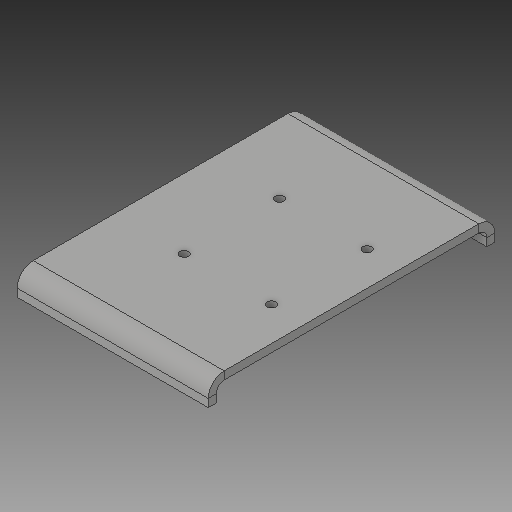
# Autodesk Inventor part: shapeoko_zplate
Saved by Autodesk Inventor 2019 (Build 230136000, 136)
## iProperties
Created: 2017-12-20
Part Number: shapeoko_zplate
Material: Generic
Document SubType Name: Sheet Metal
Designer: MISAKA
Density: 1 g/cm^3
Sheet Metal Rule: Default_mm
Appearance: Default
Author: MISAKA
Autodesk Inventor part; units mm, degrees
ref_plane "YZ Plane" through (0, 0, 0) normal (1, 0, 0) x (0, 1, 0)
ref_plane "XZ Plane" through (0, 0, 0) normal (0, 1, 0) x (-1, 0, 0)
ref_plane "XY Plane" through (0, 0, 0) normal (0, 0, 1) x (1, 0, 0)
sketch "Sketch1" plane through (0, 0, 0) normal (0, 1, 0) x (-1, 0, 0)
  line L0 (-60, 105) -> (60, 105)
  line L1 (60, 105) -> (60, 90)
  line L2 (60, -105) -> (-60, -105)
  line L3 (-60, -105) -> (-60, -90)
  line L4 (-60, 105) -> (60, -105) construction
  line L5 (60, 105) -> (-60, -105) construction
  line L6 (60, 90) -> (-60, 90)
  line L7 (60, -90) -> (-60, -90)
  line L8 (60, 90) -> (60, -90)
  line L9 (60, -90) -> (60, -105)
  line L10 (-60, -90) -> (-60, 90)
  line L11 (-60, 90) -> (-60, 105)
  line L12 (84, 0) -> (-84, 0)
  line L13 (0, -147) -> (0, 147)
  point P0 (0, 0)
  dimension "d0" = 180
  dimension "d1" = 15
  dimension "d2" = 120
  measures "d0" distance between parallel lines of L7 L6
  measures "d1" distance between parallel lines of L6 L0
  measures "d2" distance of L0.start L0.end
extrude "Plate1" add sketch "Sketch1" along normal blind 5 contours L6 L13 L12 L10 | L6 L8 L12 L13 | L12 L13 L7 L10 | L12 L8 L7 L13
sketch "Sketch2" plane through (-60, 5, 85) normal (0, 0, 1) x (1, 0, 0)
  line L0 (120, 0) -> (0, 0)
  line L1 (0, 0) -> (0, -15)
  line L2 (0, -15) -> (120, -15)
  line L3 (120, -15) -> (120, 0)
  constraints: 6 end point, 1 horizontal, 1 perpendicular, 1 vertical
edge flange "Flange1" height 15 angle 90 thickness 5 bend radius 5 thickness toward (0, 0, 1) relief tear relief width 5 relief depth 2.5 corner gap 5 corner form 0 edges at (0, 0, 90) (0, 0, -90) wall of the first edge with corners at (60, 5, 85) (-60, 5, 85) (-60, -10, 85) (60, -10, 85)
bend "Bend1"
corner "Corner1"
sketch "Sketch3" plane through (0, 0, 0) normal (0, -1, 0) x (1, 0, 0)
  circle A0 centre (-16.2613, 28.9263) radius 2.75 projected
  circle A1 centre (38.7387, 28.9263) radius 2.75 projected
  circle A2 centre (-16.2613, -31.0737) radius 2.75 projected
  circle A3 centre (38.7387, -31.0737) radius 2.75 projected
  point P0 (0, 0)
extrude "Extrusion1" cut sketch "Sketch3" against normal through all
equation "\"d3\" = Thickness"
equation "\"d4\" = BendReliefWidth"
equation "\"d5\" = BendReliefDepth"
equation "\"d6\" = MinimumRemnant"
equation "\"d7\" = TransitionRadius"
equation "\"d10\" = BendRadius"
equation "\"d11\" = CornerReliefSize"
equation "\"d12\" = GapSize"
equation "\"d13\" = JacobiRadiusSize"
equation "\"BendRadius\" = Thickness"
equation "\"BendReliefWidth\" = Thickness"
equation "\"BendReliefDepth\" = 0.5 * Thickness"
equation "\"TransitionRadius\" = BendRadius"
equation "\"JacobiRadiusSize\" = BendRadius"
equation "\"GapSize\" = Thickness"
equation "\"Thickness\" = 5"
equation "\"MinimumRemnant\" = 10"
equation "\"CornerReliefSize\" = 20"
body "Solid1"
